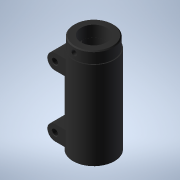
# Autodesk Inventor part: BZB-MFK
Saved by Autodesk Inventor 2021 (Build 250183000, 183)
## iProperties
Created: 2025-06-23
Part Number: BZB-MFK
Material: Generic
Catalog Web Link: www.cadenas.de
Description: base stand BZB-Accessories
Vendor: RNA
Document SubType Name: Modeling
Designer: psAdmin
Manufacturer: RNA
Mass: 318.857 g
Surface Area: 715.601 cm^2
Volume: 318.857 cm^3
Density: 1 g/cm^3
Appearance: PSOLRGB-175-175-175
Category: PARTsolutions
Company: RNA
Title: BZB-MFK
Author: Cadenas PARTsolutions
Comments: Accessories
PSOL_IDENT_0: {$CADENAS_DATA/23d-libs/rna/bunker/zubehoer/parts/bzb_muffenklemmstuesk.prj},162 {VTYP=3D},{NB=BZB-M
PSOL_IDENT_1: FK},{LINA=BZB-MFK},{NN=base stand BZB},{DATE=06.06.2017 07:14:33},{GEOMDATE=01.02.2017 10:26:24},{VE
PSOL_IDENT_2: RSION=},{LINEID=10},{WBVAR=},{WBNUMERIC=}  {NB=BZB-MFK},{LINA=BZB-MFK},{KT=DUMMY},{IDNR=BZB-MFK}
NB: BZB-MFK
NN: base stand BZB
NT: Accessories
NBSYN: $IDNR.
LINA: BZB-MFK
CATALOG: Rhein-Nadel-Automation
IDNR: BZB-MFK
SUPPLIER: RNA
ARTICLENO: BZB-MFK
BOMINFO: BZB-MFK
CREATOR: CADENAS GmbH
Autodesk Inventor part; units mm, degrees
sketch "Sketch_1" plane through (0, 0, 0) normal (0, 1, 0) x (-1, 0, 0)
  circle A0 centre (0, 0) radius 33
  constraints: 1 centre point
extrude "Extrusion1" add sketch "Sketch_1" along normal blind 140
sketch "Sketch_3" plane through (0, 0, 0) normal (0, 0, 1) x (1, 0, 0)
  arc A0 (-33, 33) -> (-33, 9) centre (-33, 21) ccw
  line L0 (-33, 9) -> (0, 9)
  line L1 (0, 9) -> (0, 33)
  line L2 (0, 33) -> (-33, 33)
  constraints: 6 end point, 2 point on circle, 1 centre point
extrude "Extrusion2" add sketch "Sketch_3" along normal mid plane 58
sketch "Sketch_4" plane through (0, 0, 0) normal (0, 0, 1) x (1, 0, 0)
  arc A0 (-33, 131) -> (-33, 107) centre (-33, 119) ccw
  line L0 (-33, 107) -> (0, 107)
  line L1 (0, 107) -> (0, 131)
  line L2 (0, 131) -> (-33, 131)
  constraints: 6 end point, 2 point on circle, 1 centre point
extrude "Extrusion3" add sketch "Sketch_4" along normal mid plane 58
sketch "Sketch4" plane through (0, 0, 0) normal (0, -1, 0) x (1, 0, 0)
  point P0 (0, 0)
hole "Hole1" at (0, 0, 0) direction (0, 1, 0) diameter 40.2 depth 140 counterbore diameter 50.2 counterbore depth 65
sketch "Sketch_5" plane through (0, 0, 0) normal (1, 0, 0) x (0, 1, 0)
  line L0 (65, 1.5) -> (0, 1.5)
  line L1 (0, 1.5) -> (0, -1.5)
  line L2 (0, -1.5) -> (65, -1.5)
  line L3 (65, -1.5) -> (65, 1.5)
  constraints: 8 end point
extrude "Extrusion4" cut sketch "Sketch_5" against normal blind 60
sketch "Sketch_6" plane through (0, 0, 0) normal (1, 0, 0) x (0, 1, 0)
  line L0 (75, 1.5) -> (75, -1.5)
  line L1 (75, -1.5) -> (140, -1.5)
  line L2 (140, -1.5) -> (140, 1.5)
  line L3 (140, 1.5) -> (75, 1.5)
  constraints: 8 end point
extrude "Extrusion5" cut sketch "Sketch_6" against normal blind 60
sketch "Sketch_7" plane through (0, 0, -29) normal (0, 0, 1) x (1, 0, 0)
  line L0 (-42.4974, 21) -> (-37.7487, 12.775)
  line L1 (-37.7487, 12.775) -> (-28.2513, 12.775)
  line L2 (-28.2513, 12.775) -> (-23.5026, 21)
  line L3 (-23.5026, 21) -> (-28.2513, 29.225)
  line L4 (-28.2513, 29.225) -> (-37.7487, 29.225)
  line L5 (-37.7487, 29.225) -> (-42.4974, 21)
  constraints: 12 end point
extrude "Extrusion6" cut sketch "Sketch_7" along normal blind 11
sketch "Sketch_8" plane through (0, 0, -29) normal (0, 0, 1) x (1, 0, 0)
  line L0 (-42.4974, 119) -> (-37.7487, 110.775)
  line L1 (-37.7487, 110.775) -> (-28.2513, 110.775)
  line L2 (-28.2513, 110.775) -> (-23.5026, 119)
  line L3 (-23.5026, 119) -> (-28.2513, 127.225)
  line L4 (-28.2513, 127.225) -> (-37.7487, 127.225)
  line L5 (-37.7487, 127.225) -> (-42.4974, 119)
  constraints: 12 end point
extrude "Extrusion7" cut sketch "Sketch_8" along normal blind 11
sketch "Sketch_9" plane through (-33, 0, 0) normal (1, 0, 0) x (0, 0, -1)
  line L0 (18, 21) -> (-29, 21)
  line L1 (-29, 21) -> (-29, 26)
  line L2 (-29, 26) -> (-28.188, 25.188)
  line L3 (-28.188, 25.188) -> (-2.312, 25.188)
  line L4 (-2.312, 25.188) -> (-1.5, 26)
  line L5 (-1.5, 26) -> (-1.5, 26.5)
  line L6 (-1.5, 26.5) -> (18, 26.5)
  line L7 (18, 26.5) -> (18, 21)
  line L8 (18, 21) -> (-29, 21)
  constraints: 18 end point
revolve "Revolution1" cut sketch "Sketch_9" angle 360 about axis through (-33, 21, -18) along (0, 0, -1)
thread "Thread1" size "M10x1.5" class "6H" standard "ISO Metric profile" full length
sketch "Sketch_10" plane through (-33, 0, 0) normal (1, 0, 0) x (0, 0, -1)
  line L0 (18, 119) -> (-29, 119)
  line L1 (-29, 119) -> (-29, 124)
  line L2 (-29, 124) -> (-28.188, 123.188)
  line L3 (-28.188, 123.188) -> (-2.312, 123.188)
  line L4 (-2.312, 123.188) -> (-1.5, 124)
  line L5 (-1.5, 124) -> (-1.5, 124.5)
  line L6 (-1.5, 124.5) -> (18, 124.5)
  line L7 (18, 124.5) -> (18, 119)
  line L8 (18, 119) -> (-29, 119)
  constraints: 18 end point
revolve "Revolution2" cut sketch "Sketch_10" angle 360 about axis through (-33, 119, -18) along (0, 0, -1)
thread "Thread2" size "M10x1.5" class "6H" standard "ISO Metric profile" full length
sketch "Sketch_11" plane through (-33, 0, 0) normal (1, 0, 0) x (0, 0, -1)
  line L0 (28, 119) -> (-17, 119)
  line L1 (-17, 119) -> (-17, 123)
  line L2 (-17, 123) -> (-16, 124)
  line L3 (-16, 124) -> (18, 124)
  line L4 (18, 124) -> (18, 127)
  line L5 (18, 127) -> (27.5, 127)
  arc A0 (28, 126.5) -> (27.5, 127) centre (27.5, 126.5) ccw
  line L6 (28, 126.5) -> (28, 119)
  line L7 (28, 119) -> (-17, 119)
  constraints: 16 end point, 2 point on circle, 1 centre point
revolve "Revolution3" add sketch "Sketch_11" angle 360 about axis through (-33, 119, -28) along (0, 0, -1)
sketch "Sketch_12" plane through (-33, 0, 0) normal (1, 0, 0) x (0, 0, -1)
  line L0 (28, 21) -> (-17, 21)
  line L1 (-17, 21) -> (-17, 25)
  line L2 (-17, 25) -> (-16, 26)
  line L3 (-16, 26) -> (18, 26)
  line L4 (18, 26) -> (18, 29)
  line L5 (18, 29) -> (27.5, 29)
  arc A0 (28, 28.5) -> (27.5, 29) centre (27.5, 28.5) ccw
  line L6 (28, 28.5) -> (28, 21)
  line L7 (28, 21) -> (-17, 21)
  constraints: 16 end point, 2 point on circle, 1 centre point
revolve "Revolution4" add sketch "Sketch_12" angle 360 about axis through (-33, 21, -28) along (0, 0, -1)
sketch "Sketch_13" plane through (-33, 21, -28) normal (0, 0, -1) x (0, 1, 0)
  line L0 (-4, -2.3094) -> (0, -4.6188)
  line L1 (0, -4.6188) -> (4, -2.3094)
  line L2 (4, -2.3094) -> (4, 2.3094)
  line L3 (4, 2.3094) -> (0, 4.6188)
  line L4 (0, 4.6188) -> (-4, 2.3094)
  line L5 (-4, 2.3094) -> (-4, -2.3094)
  constraints: 12 end point
extrude "Extrusion8" cut sketch "Sketch_13" against normal blind 4
sketch "Sketch_14" plane through (-33, 119, -28) normal (0, 0, -1) x (0, 1, 0)
  line L0 (-4, -2.3094) -> (0, -4.6188)
  line L1 (0, -4.6188) -> (4, -2.3094)
  line L2 (4, -2.3094) -> (4, 2.3094)
  line L3 (4, 2.3094) -> (0, 4.6188)
  line L4 (0, 4.6188) -> (-4, 2.3094)
  line L5 (-4, 2.3094) -> (-4, -2.3094)
  constraints: 12 end point
extrude "Extrusion9" cut sketch "Sketch_14" against normal blind 4
sketch "Sketch_15" plane through (0, 0, 0) normal (0, 0, 1) x (1, 0, 0)
  line L0 (0, 140) -> (0, 158)
  line L1 (20.25, 158) -> (20.25, 140)
  line L2 (20.25, 140) -> (31.5, 140)
  line L3 (31.5, 140) -> (31.5, 156.5)
  line L4 (31.5, 156.5) -> (30, 158)
  line L5 (30, 158) -> (20.25, 158)
  constraints: 12 end point
revolve "Revolution5" add sketch "Sketch_15" angle 360 about axis through (0, 140, 0) along (0, -1, 0)
sketch "Sketch_16" plane through (0, 0, 0) normal (0, 0, 1) x (1, 0, 0)
  circle A0 centre (0, 149) radius 4.25
  constraints: 1 centre point
extrude "Extrusion10" cut sketch "Sketch_16" along normal blind 50
ref_plane "KLEMM_XY" through (0, 65, 0) normal (0, 1, 0) x (1, 0, 0)
ref_plane "KLEMM_YZ" through (0, 65, 0) normal (1, 0, 0) x (0, 0, -1)
ref_plane "KLEMM_ZX" through (0, 65, 0) normal (0, 0, -1) x (0, 1, 0)
ref_plane "PROFIL_UP_XY" through (0, 0, 0) normal (0, -1, 0) x (1, 0, 0)
ref_plane "PROFIL_UP_YZ" through (0, 0, 0) normal (1, 0, 0) x (0, 0, 1)
ref_plane "PROFIL_UP_ZX" through (0, 0, 0) normal (0, 0, 1) x (0, -1, 0)
body "Solid1"
